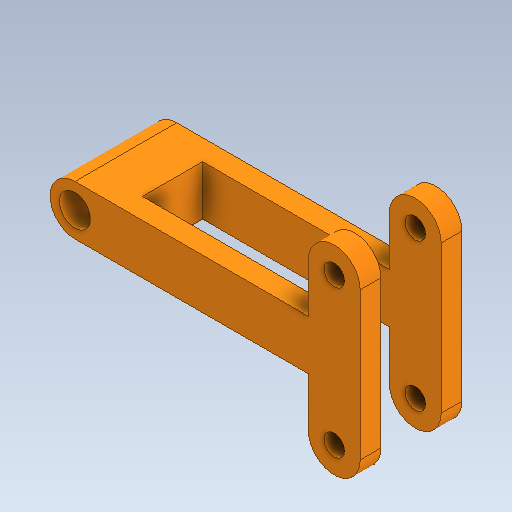
# Autodesk Inventor part: PistonPivotTop
Saved by Autodesk Inventor 2020 (Build 240168000, 168)
## iProperties
Created: 2020-09-14
Part Number: PistonPivotTop
Material: Generic
Document SubType Name: Modeling
Designer: Turing
Density: 1 g/cm^3
Appearance: Orange
Mass: 0.904919 g
Surface Area: 13.5094 cm^2
Volume: 0.904919 cm^3
Author: Turing
Autodesk Inventor part; units mm, degrees
ref_plane "YZ Plane" through (0, 0, 0) normal (1, 0, 0) x (0, 1, 0)
ref_plane "XZ Plane" through (0, 0, 0) normal (0, 1, 0) x (-1, 0, 0)
ref_plane "XY Plane" through (0, 0, 0) normal (0, 0, 1) x (1, 0, 0)
sketch "Sketch1" plane through (0, 0, 0) normal (0, 0, 1) x (1, 0, 0)
  line L0 (0, 0) -> (0, 7.105)
  line L1 (0, 0) -> (0, -7.105)
  line L2 (0, -7.105) -> (-5, -7.105)
  line L3 (-5, -7.105) -> (-5, 7.105)
  line L4 (0, 7.105) -> (-5, 7.105)
  circle A0 centre (-2.5, -7.105) radius 2.5
  circle A1 centre (-2.5, 7.105) radius 2.5
  circle A2 centre (-2.5, -7.105) radius 1
  circle A3 centre (-2.5, 7.105) radius 1
  line L5 (-5, 0) -> (-5, 2.4)
  line L6 (-5, 2.4) -> (-25.5, 2.4)
  line L7 (-25.5, 2.4) -> (-25.5, -2.4)
  line L8 (-25.5, -2.4) -> (-5, -2.4)
  dimension "d0" = 7.105
  dimension "d1" = 7.105
  dimension "d2" = 5
  dimension "d3" = 5
  dimension "d4" = 5
  dimension "d5" = 2
  dimension "d6" = 2
  dimension "d7" = 2.4
  dimension "d8" = 20.5
  dimension "d9" = 4.8
  constraints: 18 end point, 4 centre point, 4 horizontal, 3 midpoint, 2 coincident, 2 perpendicular, 2 point on line, 2 vertical
  measures "d0" distance of L0.start L0.end
  measures "d1" distance of L0.start L1.end
  measures "d2" distance of L1.end L2.end
  measures "d3" diameter of A0
  measures "d4" diameter of A1
  measures "d5" diameter of A2
  measures "d6" diameter of A3
  measures "d7" distance of L5.start L5.end
  measures "d8" distance of L5.end L6.end
  measures "d9" distance of L6.end L7.end
extrude "Extrusion1" add sketch "Sketch1" against normal blind 2 contours L1 A0 L3 A1 L0 | A1 L4 A3 | L4 A3 A1 | A0 L2 A2 | L2 A2 A0 | L3 L8 L7 L6
sketch "Sketch2" plane through (0, 0, -2) normal (0, 0, -1) x (-1, 0, 0)
  line L0 (0, 7.105) -> (0, -7.105) projected
  arc A0 (0, -7.105) -> (5, -7.105) centre (2.5, -7.105) ccw projected
  line L1 (5, -7.105) -> (5, -2.4) projected
  line L2 (5, -2.4) -> (25.5, -2.4) projected
  line L3 (25.5, -2.4) -> (25.5, 2.4) projected
  line L4 (25.5, 2.4) -> (5, 2.4) projected
  line L5 (5, 2.4) -> (5, 7.105) projected
  arc A1 (5, 7.105) -> (0, 7.105) centre (2.5, 7.105) ccw projected
  circle A2 centre (2.5, -7.105) radius 1 projected
  circle A3 centre (2.5, 7.105) radius 1 projected
  line L6 (23, 2.4) -> (25.5, 2.4)
  line L7 (25.5, 2.4) -> (25.5, -2.4)
  line L8 (25.5, -2.4) -> (23, -2.4)
  line L9 (23, -2.4) -> (23, 2.4)
  point P0 (0, 0)
  point P1 (23, -2.4)
  dimension "d26" = 2.5
  constraints: 8 end point, 2 parallel, 1 horizontal, 1 perpendicular, 1 point on line
  measures "d26" distance of L2.end L8.end
extrude "Extrusion2" add sketch "Sketch2" along normal blind 2.905 contours L4 L3 L2 L9
sketch "Sketch4" plane through (0, 0, 0) normal (0, 0, 1) x (1, 0, 0)
  arc A0 (0, 7.105) -> (-5, 7.105) centre (-2.5, 7.105) ccw projected
  line L0 (-5, 7.105) -> (-5, 2.4) projected
  line L1 (-5, 2.4) -> (-25.5, 2.4) projected
  line L2 (-25.5, 2.4) -> (-25.5, -2.4) projected
  line L3 (-25.5, -2.4) -> (-5, -2.4) projected
  line L4 (-5, -2.4) -> (-5, -7.105) projected
  arc A1 (-5, -7.105) -> (0, -7.105) centre (-2.5, -7.105) ccw projected
  line L5 (0, -7.105) -> (0, 7.105) projected
  circle A2 centre (-2.5, -7.105) radius 1 projected
  circle A3 centre (-2.5, 7.105) radius 1 projected
  line L6 (-25.5, 0) -> (-27.5, 0)
  circle A4 centre (-27.5, 0) radius 1.5
  circle A5 centre (-27.5, 0) radius 2.4
  line L7 (-25.5, -2.4) -> (-27.5, -2.4)
  line L8 (-25.5, 2.4) -> (-27.5, 2.4)
  point P0 (0, 0)
  dimension "d21" = 2
  dimension "d22" = 3
  dimension "d23" = 4.8
  constraints: 6 end point, 2 centre point, 2 coincident, 2 point on circle, 1 horizontal, 1 midpoint, 1 parallel, 1 tangent
  measures "d21" distance of L6.start L6.end
  measures "d22" diameter of A4
  measures "d23" diameter of A5
extrude "Extrusion4" add sketch "Sketch4" against normal up to surface (4.905 mm away) contours L2 A5 L8 | L2 A5 | L7 A5 L2 picked at (-25.6812, 0.5619)
mirror "Mirror2" about plane through (-24.25, 0, -4.905) normal (0, 0, -1) of "Extrusion1", "Extrusion2", "Extrusion4"
equation "\"d1\" = d0"
equation "\"d3\" = d2"
equation "\"d4\" = d2"
equation "\"d6\" = d5"
equation "\"d9\" = 2 * d7"
body "Solid1"
